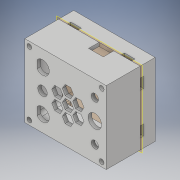
# Autodesk Inventor part: HC_box_v2
Saved by Autodesk Inventor 2018 (Build 220112000, 112)
## iProperties
Created: 2017-06-15
Part Number: HC_box_v2
Material: Generic
Document SubType Name: Modeling
Designer: boss
Density: 1 g/cm^3
Appearance: Default
Author: boss
Autodesk Inventor part; units mm, degrees
ref_plane "YZ Plane" through (0, 0, 0) normal (1, 0, 0) x (0, 1, 0)
ref_plane "XZ Plane" through (0, 0, 0) normal (0, 1, 0) x (-1, 0, 0)
sketch "Sketch1" plane through (0, 0, 0) normal (0, 0, 1) x (1, 0, 0)
  line L0 (-29.591, -26.416) -> (29.591, -26.416)
  line L1 (29.591, -26.416) -> (29.591, 26.416)
  line L2 (29.591, 26.416) -> (-29.591, 26.416)
  line L3 (-29.591, 26.416) -> (-29.591, -26.416)
  line L4 (-29.591, -26.416) -> (29.591, 26.416) construction
  line L5 (29.591, -26.416) -> (-29.591, 26.416) construction
  point P0 (0, 0)
  dimension "d0" = 59.182
  dimension "d1" = 52.832
  constraints: 12 end point, 2 midpoint, 2 parallel, 1 horizontal, 1 perpendicular
  measures "d0" distance of L2.end L1.end
  measures "d1" distance of L1.end L0.end
extrude "Extrusion1" add sketch "Sketch1" along normal blind 2.54
sketch "Sketch2" plane through (0, 0, 2.54) normal (0, 0, 1) x (1, 0, 0)
  line L0 (-27.051, -23.876) -> (27.051, -23.876)
  line L1 (27.051, -23.876) -> (27.051, 23.876)
  line L2 (27.051, 23.876) -> (-27.051, 23.876)
  line L3 (-27.051, 23.876) -> (-27.051, -23.876)
  line L4 (-27.051, -23.876) -> (27.051, 23.876) construction
  line L5 (27.051, -23.876) -> (-27.051, 23.876) construction
  line L6 (29.591, 26.416) -> (-29.591, 26.416) projected
  line L7 (29.591, -26.416) -> (29.591, 26.416) projected
  line L8 (-29.591, -26.416) -> (29.591, -26.416)
  line L9 (29.591, -26.416) -> (29.591, 26.416)
  line L10 (29.591, 26.416) -> (-29.591, 26.416)
  line L11 (-29.591, 26.416) -> (-29.591, -26.416)
  line L12 (-29.591, -26.416) -> (29.591, 26.416) construction
  line L13 (29.591, -26.416) -> (-29.591, 26.416) construction
  line L14 (25.7048, 21.971) -> (-25.7048, 21.971) construction
  line L15 (-25.7048, 21.971) -> (-25.7048, -21.971) construction
  line L16 (-25.7048, -21.971) -> (25.7048, -21.971) construction
  line L17 (25.7048, -21.971) -> (25.7048, 21.971) construction
  line L18 (25.7048, 21.971) -> (-25.7048, -21.971) construction
  line L19 (-25.7048, 21.971) -> (25.7048, -21.971) construction
  point P0 (0, 0)
  dimension "d4" = 2.54
  dimension "d5" = 2.54
  dimension "d39" = 51.4096
  dimension "d40" = 43.942
  constraints: 36 end point, 6 midpoint, 6 parallel, 3 horizontal, 3 perpendicular
  measures "d4" distance between parallel lines of L6 L2
  measures "d5" distance between parallel lines of L7 L1
  measures "d39" distance of L16.end L15.end
  measures "d40" distance of L15.end L14.end
extrude "Extrusion2" add sketch "Sketch2" along normal blind 30.48
sketch "Sketch3" plane through (-29.591, 26.416, 0) normal (0, 1, 0) x (1, 0, 0)
  line L0 (40.005, -10.922) -> (29.337, -10.922)
  line L1 (29.337, -10.922) -> (29.337, -18.542)
  line L2 (29.337, -18.542) -> (40.005, -18.542)
  line L3 (40.005, -18.542) -> (40.005, -10.922)
  line L4 (40.005, -10.922) -> (29.337, -18.542) construction
  line L5 (29.337, -10.922) -> (40.005, -18.542) construction
  line L6 (59.182, 0) -> (0, 0) projected
  line L7 (0, 0) -> (0, -33.02) projected
  line L8 (29.591, 0) -> (29.591, -33.02) construction
  line L9 (56.642, -33.02) -> (2.54, -33.02) construction
  point P0 (34.671, -14.732)
  dimension "d10" = 5.08
  dimension "d11" = 10.668
  dimension "d12" = 7.62
  dimension "d44" = 14.732
  constraints: 14 end point, 3 midpoint, 2 parallel, 1 horizontal, 1 perpendicular
  measures "d10" distance from line of L8 point (34.671, -14.732)
  measures "d11" distance of L1.end L2.end
  measures "d12" distance of L0.end L1.end
  measures "d44" distance from line of L6 point (34.671, -14.732)
extrude "Extrusion3" cut sketch "Sketch3" against normal up to surface (2.54 mm away)
ref_plane "Work Plane1" through (0, 0, 10.922) normal (0, 0, 1) x (1, 0, 0)
sketch "Sketch4" plane through (0, 0, 33.02) normal (0, 0, 1) x (1, 0, 0)
  line L0 (29.591, 26.416) -> (-29.591, 26.416) projected
  line L1 (29.591, -26.416) -> (-29.591, -26.416)
  line L2 (-29.591, -26.416) -> (-29.591, 26.416)
  line L3 (-29.591, 26.416) -> (29.591, 26.416)
  line L4 (29.591, 26.416) -> (29.591, -26.416)
  line L5 (29.591, -26.416) -> (-29.591, 26.416) construction
  line L6 (-29.591, -26.416) -> (29.591, 26.416) construction
  point P0 (0, 0)
  constraints: 12 end point, 2 midpoint, 2 parallel, 1 horizontal, 1 perpendicular
extrude "Extrusion4" add sketch "Sketch4" along normal blind 2.54
sketch "Sketch5" plane through (0, 0, 35.56) normal (0, 0, 1) x (1, 0, 0)
  circle A0 centre (-16.6948, 14.7623) radius 4.8895
  line L0 (13.97, 21.59) -> (-3.81, 21.59)
  line L1 (-3.81, 21.59) -> (-3.81, -21.59)
  line L2 (-3.81, -21.59) -> (13.97, -21.59)
  line L3 (13.97, -21.59) -> (13.97, 21.59)
  line L4 (13.97, 21.59) -> (-3.81, -21.59) construction
  line L5 (-3.81, 21.59) -> (13.97, -21.59) construction
  line L6 (-46.5157, 0) -> (71.9571, 0) projected
  circle A1 centre (-16.6948, 0) radius 3.429
  line L7 (-20.6953, 11.951) -> (-20.6953, 17.5735)
  circle A2 centre (-16.6948, -14.7623) radius 4.8895
  line L8 (-20.6953, -11.951) -> (-20.6953, -17.5735)
  circle A3 centre (21.3137, 14.7623) radius 2.667
  circle A4 centre (21.3137, -14.7623) radius 2.667
  circle A5 centre (21.3137, 0) radius 4.8895
  point P0 (0, 0)
  point P1 (5.08, 0)
  dimension "d18" = 9.779
  dimension "d19" = 17.78
  dimension "d21" = 6.858
  dimension "d22" = 8.89
  dimension "d23" = 5.334
  dimension "d41" = 43.18
  dimension "d42" = 5.08
  dimension "d103" = 9.779
  constraints: 16 end point, 6 centre point, 4 point on circle, 4 symmetric about line, 3 point on line, 2 midpoint, 2 parallel, 1 horizontal, 1 perpendicular, 1 vertical, 2 other
  measures "d18" diameter of A0
  measures "d19" distance of L2.end L1.end
  measures "d21" diameter of A1
  measures "d23" diameter of A3
  measures "d41" distance of L2.end L0.start
  measures "d42" distance of point (0, 0) point (5.08, 0)
  measures "d103" diameter of A5
extrude "Extrusion5" cut sketch "Sketch5" against normal blind 2.54 contours A0 L7 | A1 L6 | L6 A1 | A5 L6 | L6 A5 | A2 L8 | A3 | A4 picked at (-15.9328, 15.8566) picked at (-15.3105, -13.9389)
sketch "Sketch6" plane through (0, 0, 2.54) normal (0, 0, 1) x (1, 0, 0)
  circle A0 centre (0, -17.78) radius 1.7272
  line L0 (-41.4274, 0) -> (41.4274, 0) projected
  circle A1 centre (0, 17.78) radius 1.7272
  point P0 (0, 0)
  dimension "d26" = 3.4544
  dimension "d27" = 35.56
  constraints: 2 centre point, 1 symmetric about line, 1 other
  measures "d26" diameter of A0
  measures "d27" distance of A1.centre A0.centre
extrude "Extrusion6" cut sketch "Sketch6" against normal blind 2.54
sketch "Sketch7" plane through (0, 0, 35.56) normal (0, 0, 1) x (1, 0, 0)
  line L0 (-29.591, 26.416) -> (-29.591, -26.416) projected
  line L1 (-29.591, -26.416) -> (29.591, -26.416) projected
  line L2 (-46.5157, 0) -> (71.9571, 0) projected
  line L3 (0, 36.9824) -> (0, -36.9824) projected
  point P0 (0, 0)
  point P1 (-26.289, -23.114)
  point P2 (-26.289, 23.114)
  point P3 (26.289, -23.114)
  point P4 (26.289, 23.114)
  dimension "d30" = 3.302
  dimension "d31" = 3.302
  constraints: 3 symmetric about line
  measures "d30" distance from line of L0 point (-26.289, -23.114)
  measures "d31" distance from line of L1 point (-26.289, -23.114)
hole "Hole1" at (-26.289, -23.114, 35.56) at (26.289, -23.114, 35.56) at (26.289, 23.114, 35.56) at (-26.289, 23.114, 35.56) direction (0, 0, -1) diameter 3.4544 end through all clearance for "Flat Head Machine Screw (82)" size "#5" standard "Ansi Unified Screw Threads"
sketch "Sketch9" plane through (-29.591, -26.416, 0) normal (-1, 0, 0) x (0, 0, 1)
  line L0 (8.382, 45.212) -> (10.922, 45.212)
  line L1 (10.922, 45.212) -> (10.922, 37.592)
  line L2 (10.922, 37.592) -> (8.382, 37.592)
  line L3 (8.382, 37.592) -> (8.382, 45.212)
  line L4 (8.382, 45.212) -> (10.922, 37.592) construction
  line L5 (10.922, 45.212) -> (8.382, 37.592) construction
  line L6 (0, 52.832) -> (0, 0) projected
  line L7 (-7.112, 26.416) -> (42.672, 26.416) projected
  line L8 (8.382, 7.62) -> (10.922, 7.62)
  line L9 (10.922, 7.62) -> (10.922, 15.24)
  line L10 (10.922, 15.24) -> (8.382, 15.24)
  line L11 (8.382, 15.24) -> (8.382, 7.62)
  line L12 (8.382, 7.62) -> (10.922, 15.24) construction
  line L13 (10.922, 7.62) -> (8.382, 15.24) construction
  line L14 (0, 52.832) -> (35.56, 52.832) projected
  point P0 (0, 26.416)
  point P1 (9.652, 41.402)
  point P2 (9.652, 11.43)
  dimension "d45" = 2.54
  dimension "d46" = 7.62
  dimension "d47" = 10.922
  dimension "d57" = 7.62
  constraints: 24 end point, 5 symmetric about line, 4 midpoint, 2 parallel, 1 horizontal, 1 perpendicular
  measures "d45" distance of L1.end L2.end
  measures "d46" distance of L0.end L1.end
  measures "d47" distance between parallel lines of L6 L1
  measures "d57" distance between parallel lines of L14 L0
extrude "Extrusion7" cut sketch "Sketch9" against normal through all
sketch "Sketch10" plane through (-29.591, 26.416, 0) normal (0, 1, 0) x (1, 0, 0)
  line L0 (52.832, -8.382) -> (45.212, -8.382)
  line L1 (45.212, -8.382) -> (45.212, -10.922)
  line L2 (45.212, -10.922) -> (52.832, -10.922)
  line L3 (52.832, -10.922) -> (52.832, -8.382)
  line L4 (52.832, -8.382) -> (45.212, -10.922) construction
  line L5 (45.212, -8.382) -> (52.832, -10.922) construction
  line L6 (59.182, 0) -> (0, 0) projected
  line L7 (29.591, 7.112) -> (29.591, -42.672) projected
  line L8 (6.35, -8.382) -> (13.97, -8.382)
  line L9 (13.97, -8.382) -> (13.97, -10.922)
  line L10 (13.97, -10.922) -> (6.35, -10.922)
  line L11 (6.35, -10.922) -> (6.35, -8.382)
  line L12 (6.35, -8.382) -> (13.97, -10.922) construction
  line L13 (13.97, -8.382) -> (6.35, -10.922) construction
  line L14 (59.182, 0) -> (59.182, -35.56) projected
  point P0 (29.591, 0)
  point P1 (49.022, -9.652)
  point P2 (10.16, -9.652)
  dimension "d52" = 7.62
  dimension "d53" = 2.54
  dimension "d54" = 10.922
  dimension "d58" = 6.35
  constraints: 24 end point, 5 symmetric about line, 4 midpoint, 2 parallel, 1 horizontal, 1 perpendicular
  measures "d52" distance of L2.end L1.end
  measures "d53" distance of L1.end L0.end
  measures "d54" distance between parallel lines of L6 L2
  measures "d58" distance between parallel lines of L14 L3
extrude "Extrusion8" cut sketch "Sketch10" against normal through all
sketch "Sketch12" plane through (0, 0, 35.56) normal (0, 0, 1) x (1, 0, 0)
  line L0 (-2.3059, 0) -> (-0.2739, 3.5195)
  line L1 (-0.2739, 3.5195) -> (3.7901, 3.5195)
  line L2 (3.7901, 3.5195) -> (5.8221, 0)
  line L3 (5.8221, 0) -> (3.7901, -3.5195)
  line L4 (3.7901, -3.5195) -> (-0.2739, -3.5195)
  line L5 (-0.2739, -3.5195) -> (-2.3059, 0)
  line L6 (-3.3219, 0) -> (-0.7819, 4.3994)
  line L7 (-0.7819, 4.3994) -> (4.2981, 4.3994)
  line L8 (4.2981, 4.3994) -> (6.8381, 0)
  line L9 (6.8381, 0) -> (4.2981, -4.3994)
  line L10 (4.2981, -4.3994) -> (-0.7819, -4.3994)
  line L11 (-0.7819, -4.3994) -> (-3.3219, 0)
  line L12 (-41.4274, 0) -> (41.4274, 0) projected
  line L13 (-2.3059, 8.7988) -> (-0.2739, 12.3183)
  line L14 (-0.2739, 12.3183) -> (3.7901, 12.3183)
  line L15 (3.7901, 12.3183) -> (5.8221, 8.7988)
  line L16 (5.8221, 8.7988) -> (3.7901, 5.2793)
  line L17 (3.7901, 5.2793) -> (-0.2739, 5.2793)
  line L18 (-0.2739, 5.2793) -> (-2.3059, 8.7988)
  line L19 (-3.3219, 8.7988) -> (-0.7819, 13.1982)
  line L20 (-0.7819, 13.1982) -> (4.2981, 13.1982)
  line L21 (4.2981, 13.1982) -> (6.8381, 8.7988)
  line L22 (6.8381, 8.7988) -> (4.2981, 4.3994)
  line L23 (4.2981, 4.3994) -> (-0.7819, 4.3994)
  line L24 (-0.7819, 4.3994) -> (-3.3219, 8.7988)
  line L25 (-1.7979, 4.3994) -> (-3.8299, 0.8799)
  line L26 (-3.3219, 0) -> (-8.4019, 0)
  line L27 (-3.8299, 7.9189) -> (-1.7979, 4.3994)
  line L28 (-3.8299, 0.8799) -> (-7.8939, 0.8799)
  line L29 (-7.8939, 0.8799) -> (-9.9259, 4.3994)
  line L30 (-8.4019, 0) -> (-10.9419, 4.3994)
  line L31 (-9.9259, 4.3994) -> (-7.8939, 7.9189)
  line L32 (-10.9419, 4.3994) -> (-8.4019, 8.7988)
  line L33 (-7.8939, 7.9189) -> (-3.8299, 7.9189)
  line L34 (-8.4019, 8.7988) -> (-3.3219, 8.7988)
  line L35 (-3.3219, 8.7988) -> (-0.7819, 4.3994)
  line L36 (-3.3219, 0) -> (-0.7819, 4.3994)
  line L37 (-3.8299, -0.8799) -> (-1.7979, -4.3994)
  line L38 (-0.7819, -4.3994) -> (-3.3219, -8.7988)
  line L39 (-7.8939, -0.8799) -> (-3.8299, -0.8799)
  line L40 (-1.7979, -4.3994) -> (-3.8299, -7.9189)
  line L41 (-3.8299, -7.9189) -> (-7.8939, -7.9189)
  line L42 (-3.3219, -8.7988) -> (-8.4019, -8.7988)
  line L43 (-7.8939, -7.9189) -> (-9.9259, -4.3994)
  line L44 (-8.4019, -8.7988) -> (-10.9419, -4.3994)
  line L45 (-9.9259, -4.3994) -> (-7.8939, -0.8799)
  line L46 (-10.9419, -4.3994) -> (-8.4019, 0)
  line L47 (-8.4019, 0) -> (-3.3219, 0)
  line L48 (-0.7819, -4.3994) -> (-3.3219, 0)
  line L49 (-0.2739, -5.2793) -> (3.7901, -5.2793)
  line L50 (4.2981, -4.3994) -> (6.8381, -8.7988)
  line L51 (-2.3059, -8.7988) -> (-0.2739, -5.2793)
  line L52 (3.7901, -5.2793) -> (5.8221, -8.7988)
  line L53 (5.8221, -8.7988) -> (3.7901, -12.3183)
  line L54 (6.8381, -8.7988) -> (4.2981, -13.1982)
  line L55 (3.7901, -12.3183) -> (-0.2739, -12.3183)
  line L56 (4.2981, -13.1982) -> (-0.7819, -13.1982)
  line L57 (-0.2739, -12.3183) -> (-2.3059, -8.7988)
  line L58 (-0.7819, -13.1982) -> (-3.3219, -8.7988)
  line L59 (-3.3219, -8.7988) -> (-0.7819, -4.3994)
  line L60 (4.2981, -4.3994) -> (-0.7819, -4.3994)
  line L61 (5.3141, -4.3994) -> (7.3461, -0.8799)
  line L62 (6.8381, 0) -> (11.9181, 0)
  line L63 (7.3461, -7.9189) -> (5.3141, -4.3994)
  line L64 (7.3461, -0.8799) -> (11.4101, -0.8799)
  line L65 (11.4101, -0.8799) -> (13.4421, -4.3994)
  line L66 (11.9181, 0) -> (14.4581, -4.3994)
  line L67 (13.4421, -4.3994) -> (11.4101, -7.9189)
  line L68 (14.4581, -4.3994) -> (11.9181, -8.7988)
  line L69 (11.4101, -7.9189) -> (7.3461, -7.9189)
  line L70 (11.9181, -8.7988) -> (6.8381, -8.7988)
  line L71 (6.8381, -8.7988) -> (4.2981, -4.3994)
  line L72 (6.8381, 0) -> (4.2981, -4.3994)
  line L73 (7.3461, 0.8799) -> (5.3141, 4.3994)
  line L74 (4.2981, 4.3994) -> (6.8381, 8.7988)
  line L75 (11.4101, 0.8799) -> (7.3461, 0.8799)
  line L76 (5.3141, 4.3994) -> (7.3461, 7.9189)
  line L77 (7.3461, 7.9189) -> (11.4101, 7.9189)
  line L78 (6.8381, 8.7988) -> (11.9181, 8.7988)
  line L79 (11.4101, 7.9189) -> (13.4421, 4.3994)
  line L80 (11.9181, 8.7988) -> (14.4581, 4.3994)
  line L81 (13.4421, 4.3994) -> (11.4101, 0.8799)
  line L82 (14.4581, 4.3994) -> (11.9181, 0)
  line L83 (11.9181, 0) -> (6.8381, 0)
  line L84 (4.2981, 4.3994) -> (6.8381, 0)
  point P0 (1.7581, 0)
  point P1 (1.7581, 0)
  point P2 (1.7581, 8.7988)
  point P3 (1.7581, 8.7988)
  point P4 (-5.8619, 4.3994)
  point P5 (-5.8619, 4.3994)
  point P6 (-5.8619, -4.3994)
  point P7 (-5.8619, -4.3994)
  point P8 (1.7581, -8.7988)
  point P9 (1.7581, -8.7988)
  point P10 (9.3781, -4.3994)
  point P11 (9.3781, -4.3994)
  point P12 (9.3781, 4.3994)
  point P13 (9.3781, 4.3994)
  dimension "d87" = 4.064
  dimension "d88" = 5.08
  dimension "d89" = 4.064
  dimension "d90" = 5.08
  dimension "d93" = 360
  dimension "d100" = 13.1982
  dimension "d101" = 8.7988
  constraints: 168 end point, 7 coincident, 4 horizontal, 1 point on line, 221 other
  measures "d87" distance of L0.start point (1.758, 0)
  measures "d88" distance of L6.start point (1.758, 0)
  measures "d89" distance of L13.start point (1.758, 8.799)
  measures "d90" distance of L19.start point (1.758, 8.799)
  measures "d100" distance between parallel lines of L20 L12
  measures "d101" distance between parallel lines of L38 L82
extrude "Extrusion9" cut sketch "Sketch12" against normal blind 25.4 contours L12 L3 L4 L5 | L0 L1 L2 L12 | L13 L14 L15 L16 L17 L18 | L25 L28 L29 L31 L33 L27 | L37 L40 L41 L43 L45 L39 | L49 L52 L53 L55 L57 L51 | L61 L64 L65 L67 L69 L63 | L73 L76 L77 L79 L81 L75
split body "Split3" result two bodies by plane through (0, 0, 10.922) normal (0, 0, 1) first body at (-25.1816, 0, 35.06)
body "Solid6"
body "Solid7"
